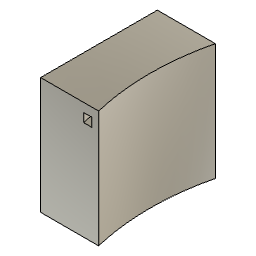
mount (Autodesk Fusion 360 design; units mm, degrees)
Autodesk Fusion 360 part; units mm, degrees
sketch "Sketch1" plane through (0, 0, 0) normal (0, 0, 1) x (1, 0, 0)
  line L0 (0, 0) -> (0, 80)
  line L1 (0, 80) -> (35, 80)
  line L2 (35, 80) -> (35, 0)
  line L3 (35, 0) -> (0, 0)
  line L4 (35, 40) -> (205, 40)
  circle A0 centre (205, 40) radius 170
  line L5 (35, 80) -> (48, 80)
  line L6 (35, 0) -> (60.4996, 0)
  circle A1 centre (205, 40) radius 174
  circle A2 centre (205, 40) radius 180
  dimension "d9" = 80
  dimension "d10" = 35
  dimension "d11" = 170
  dimension "d12" = 340
  dimension "d13" = 4
  dimension "d14" = 10
  constraint coincident L0.start L3.end
  constraint vertical L0
  constraint perpendicular L0 L1
  constraint perpendicular L1 L2
  constraint perpendicular L0 L3
  constraint midpoint L2 L4.start
  constraint perpendicular L2 L4
  constraint coincident L4.end A0.centre
  constraint perpendicular L2 L5
  constraint perpendicular L2 L6
  measures "d9" distance of L0.start L0.end
  measures "d10" distance of L0.end L1.end
  measures "d11" distance of L4.start L4.end
  measures "d12" diameter of A0
extrude "Extrude1" add sketch "Sketch1" along normal blind 12 contours L0 L1 L3 A2 | L1 L2 L3 A1 A2 | L2 L6 A1 | L2 L5 A1 | L2 A1 | L2 A0 L6 A1 | L2 A0 L5 A1 makes body 1
extrude "Extrude2" cut sketch "Sketch1" along normal blind 6 contours L1 L2 L3 A1 A2 bodies 1
extrude "Extrude3" add sketch "Sketch1" against normal blind 68 contours L0 L1 L3 A2 | L1 L2 L3 A1 A2 | L2 L6 A1 | L2 L5 A1 | L2 A1 | L2 A0 L6 A1 | L2 A0 L5 A1 bodies 1
sketch "Sketch2" plane through (0, 0, 0) normal (-1, 0, 0) x (0, -1, 0)
  line L0 (0, -68) -> (0, 12)
  line L1 (0, 12) -> (-80, 12)
  line L2 (-80, 12) -> (-80, -68)
  line L3 (-80, -68) -> (0, -68)
  line L4 (-80, 12) -> (0, -68)
  line L5 (-40, -28) -> (-23.3333, -28)
  line L6 (-40, -28) -> (-56.6667, -28)
  line L7 (-56.6667, -28) -> (-40, 0.8675)
  line L8 (-56.6667, -28) -> (-10.4786, -28) construction
  line L9 (-23.3333, -28) -> (-40, 0.8675)
  line L10 (-23.3333, -28) -> (22.8547, -28) construction
  line L11 (-40, 0.8675) -> (-15, -42.4338)
  line L12 (-40, 0.8675) -> (-65, -42.4338)
  line L13 (-65, -42.4338) -> (-15, -42.4338)
  circle A0 centre (-40, -28) radius 28.8675
  circle A1 centre (-40, 0.8675) radius 1.5
  circle A2 centre (-15, -42.4338) radius 1.5
  circle A3 centre (-65, -42.4338) radius 1.5
  circle A4 centre (-40, -28) radius 35
  dimension "d21" = 16.6667
  dimension "d22" = 16.6667
  dimension "d23" = 60
  dimension "d24" = 120
  dimension "d25" = 50
  dimension "d26" = 50
  dimension "d27" = 3
  dimension "d28" = 3
  dimension "d29" = 3
  dimension "d32" = 70
  constraint coincident L1.end L2.start
  constraint coincident L0.start L3.end
  constraint midpoint L4 L5.start
  constraint horizontal L5
  constraint parallel L5 L6
  constraint horizontal L8
  constraint horizontal L10
  constraint parallel L9 L11
  constraint parallel L7 L12
  constraint coincident L5.start L6.start
  constraint coincident L7.end A0
  constraint coincident L7.end L9.end
  constraint coincident L11.end L13.end
  constraint coincident L12.end L13.start
  constraint concentric A0 A4
  measures "d21" distance of L5.start L5.end
  measures "d22" distance of L5.start L6.end
  measures "d23" angle of L7 L8
  measures "d24" angle of L9 L10
  measures "d25" distance of L7.end L11.end
  measures "d26" distance of L7.end L12.end
  measures "d27" diameter of A1
  measures "d28" diameter of A2
  measures "d29" diameter of A3
  measures "d32" diameter of A4
extrude "Extrude4" cut sketch "Sketch2" against normal blind 30 contours A0 A3 | L13 A0 A3 | L13 A0 A2 | A0 A2 | L12 L13 A3 | L11 L13 A2 | L12 A0 A3 | L11 A0 A2 | A0 A1 | L7 L12 A0 A1 | L7 L9 L11 L12 A1 | L9 L11 A0 A1 bodies 1
extrude "Extrude5" add sketch "Sketch2" along normal blind 10 separate body contours L4 A0 A3 A4 | L4 A0 A1 A2 A4 | L4 L13 A0 A3 | L4 L13 A0 A2 | L4 L6 L12 L13 A3 | L4 L5 L11 L13 A2 | L4 L7 L12 A0 A1 | L4 L7 L12 A0 A3 | L4 L6 L7 L12 | L4 L5 L7 L9 L11 L12 A1 | L9 L11 A0 A1 A2 makes body 2
hidden bodies 2
equation "direk_radius = 170 mm"
equation "square_dimension = 80 mm"
equation "square_depth = 35 mm"
equation "d9 = square_dimension"
equation "d10 = square_depth"
equation "d11 = direk_radius"
equation "d12 = direk_radius * 2"
equation "d19 = 12 mm - square_dimension"
equation "d21 = ( ( 50 / 3 ) * 1 mm )"
equation "d22 = ( 50 / 3 ) * 1 mm"
